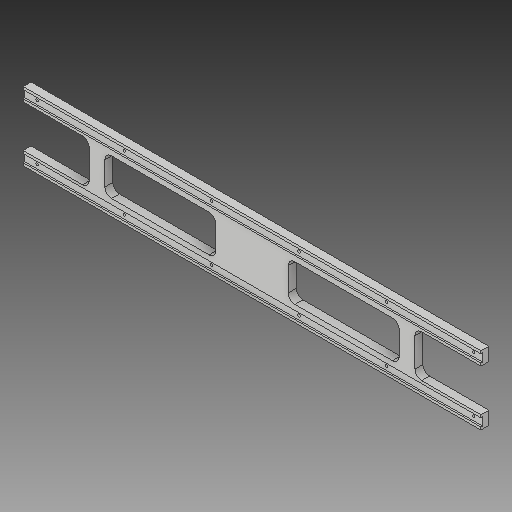
# Autodesk Inventor part: DriveTrainTop
Saved by Autodesk Inventor 2017 (Build 210142000, 142)
## iProperties
Created: 2016-10-18
Part Number: DriveTrainTop
Material: Generic
Document SubType Name: Sheet Metal
Designer: aesen
Density: 1 g/cm^3
Sheet Metal Rule: Default_mm
Appearance: Default
Author: aesen
Autodesk Inventor part; units mm, degrees
ref_plane "YZ Plane" through (0, 0, 0) normal (1, 0, 0) x (0, 1, 0)
ref_plane "XZ Plane" through (0, 0, 0) normal (0, 1, 0) x (-1, 0, 0)
ref_plane "XY Plane" through (0, 0, 0) normal (0, 0, 1) x (1, 0, 0)
sketch "Sketch1" plane through (0, 0, 0) normal (0, 0, 1) x (1, 0, 0)
  line L0 (-115.57, 41.275) -> (435.2925, 41.275)
  line L1 (435.2925, -41.275) -> (-115.57, -41.275)
  line L2 (422, 41.275) -> (422, 25.4)
  line L3 (424, -41.275) -> (424, -25.4)
  line L4 (355.9175, 17.4) -> (355.9175, -17.4)
  line L5 (355.9175, 6) -> (336.8675, 6)
  line L6 (321, 41.275) -> (321, 22.225)
  line L7 (322, -41.275) -> (322, -22.225)
  line L8 (336.8675, 14.225) -> (336.8675, -14.225)
  line L9 (-36.195, -17.4) -> (-36.195, 17.4)
  line L10 (-36.195, 0) -> (-17.145, 0)
  line L11 (-17.145, 14.225) -> (-17.145, -14.225)
  line L12 (-9.145, -22.225) -> (108.205, -22.225)
  line L13 (116.205, -14.225) -> (116.205, 14.225)
  line L14 (108.205, 22.225) -> (-9.145, 22.225)
  line L15 (116.205, 12) -> (203.518, 12)
  line L16 (211.518, 22.225) -> (328.8675, 22.225)
  line L17 (203.518, 14.225) -> (203.518, -14.225)
  line L18 (211.518, -22.225) -> (328.8675, -22.225)
  arc A0 (-9.145, 22.225) -> (-17.145, 14.225) centre (-9.145, 14.225) ccw
  arc A1 (116.205, 14.225) -> (108.205, 22.225) centre (108.205, 14.225) ccw
  arc A2 (-17.145, -14.225) -> (-9.145, -22.225) centre (-9.145, -14.225) ccw
  arc A3 (108.205, -22.225) -> (116.205, -14.225) centre (108.205, -14.225) ccw
  arc A4 (211.518, 22.225) -> (203.518, 14.225) centre (211.518, 14.225) ccw
  arc A5 (336.8675, 14.225) -> (328.8675, 22.225) centre (328.8675, 14.225) ccw
  arc A6 (328.8675, -22.225) -> (336.8675, -14.225) centre (328.8675, -14.225) ccw
  arc A7 (203.518, -14.225) -> (211.518, -22.225) centre (211.518, -14.225) ccw
  arc A8 (363.9175, 25.4) -> (355.9175, 17.4) centre (363.9175, 17.4) ccw
  arc A9 (355.9175, -17.4) -> (363.9175, -25.4) centre (363.9175, -17.4) ccw
  arc A10 (-36.195, 17.4) -> (-44.195, 25.4) centre (-44.195, 17.4) ccw
  arc A11 (-44.195, -25.4) -> (-36.195, -17.4) centre (-44.195, -17.4) ccw
  line L19 (435.2925, -41.275) -> (435.2925, 38.1)
  line L20 (-115.57, 41.275) -> (-115.57, -38.1)
  line L21 (-44.195, 25.4) -> (-115.57, 25.4)
  line L22 (-44.195, -25.4) -> (-115.57, -25.4)
  line L23 (363.9175, 25.4) -> (435.2925, 25.4)
  line L24 (363.9175, -25.4) -> (435.2925, -25.4)
  line L25 (-115.57, -38.1) -> (-115.57, -41.275)
  line L26 (435.2925, 41.275) -> (435.2925, 38.1)
  point P0 (0, 0)
  point P1 (0, 0)
  point P2 (-36.195, 25.4)
  point P3 (154, 41.275)
  point P4 (157.175, 41.275)
  point P5 (154, -41.275)
  point P6 (157.175, -41.275)
  dimension "d0" = 15.875
  dimension "d1" = 15.875
  dimension "d2" = 19.05
  dimension "d3" = 19.05
  dimension "d4" = 19.05
  dimension "d5" = 19.05
  dimension "d6" = 44.45
  dimension "d7" = 133.35
  dimension "d8" = 87.313
  dimension "d9" = 133.3495
  dimension "d10" = 8
  dimension "d11" = 79.375
  dimension "d12" = 79.375
  dimension "d13" = 550.8625
  constraints: 54 end point, 24 point on circle, 20 tangent, 15 point on line, 12 centre point, 11 equal radius, 9 perpendicular, 8 vertical, 5 horizontal, 2 parallel, 1 midpoint
  measures "d0" distance of L2.start L2.end
  measures "d1" distance of L3.end L3.start
  measures "d2" distance of L5.start L5.end
  measures "d3" distance of L6.start L6.end
  measures "d4" distance of L7.end L7.start
  measures "d5" distance of L10.start L10.end
  measures "d6" distance between parallel lines of L12 L14
  measures "d7" distance between parallel lines of L13 L11
  measures "d8" distance of L15.end L15.start
  measures "d9" distance between parallel lines of L8 L17
  measures "d10" radius of A0
  measures "d11" distance between parallel lines of L19 L4
  measures "d12" distance between parallel lines of L20 L9
  measures "d13" distance between parallel lines of L19 L20
extrude "Extrusion1" add sketch "Sketch1" along normal mid plane 9.525 contours L0 L6 L16 A4 L17 L15 L13 A1 L14 A0 L11 L10 L9 A10 L21 L20 | L0 L2 L23 A8 L4 L5 L8 A5 L16 L6 | L0 L26 L19 L23 L2 | L22 A11 L9 L10 L11 A2 L12 A3 L13 L15 L17 A7 L18 L7 L1 L25 L20 | L19 L1 L3 L24 | L5 L4 A9 L24 L3 L1 L7 L18 A6 L8
sketch "Sketch2" plane through (0, 0, 4.7625) normal (0, 0, 1) x (1, 0, 0)
  line L0 (-115.57, 41.275) -> (154, 41.275)
  line L1 (-71.7405, 41.275) -> (-71.7405, 38.1)
  line L2 (-44.195, 25.4) -> (-115.57, 25.4)
  line L3 (-83, 25.4) -> (-83, 28.575)
  line L4 (154, -41.275) -> (-130.57, -41.275)
  line L5 (-85, -41.275) -> (-85, -38.1)
  line L6 (-115.57, -25.4) -> (-44.195, -25.4)
  line L7 (-76, -25.4) -> (-76, -28.575)
  line L8 (-115.57, 25.4) -> (-115.57, 41.275)
  line L9 (435.2925, 25.4) -> (435.2925, 38.1)
  line L10 (-115.57, 38.1) -> (435.2925, 38.1)
  line L11 (435.2925, 38.1) -> (435.2925, 28.575)
  line L12 (435.2925, 28.575) -> (-115.57, 28.575)
  line L13 (-115.57, 28.575) -> (-115.57, 38.1)
  line L14 (-115.57, -38.1) -> (-115.57, -25.4)
  line L15 (435.2925, -25.4) -> (435.2925, -41.275)
  line L16 (-115.57, -28.575) -> (435.2925, -28.575)
  line L17 (435.2925, -28.575) -> (435.2925, -38.1)
  line L18 (435.2925, -38.1) -> (-115.57, -38.1)
  line L19 (-115.57, -38.1) -> (-115.57, -28.575)
  point P0 (0, 0)
  point P1 (0, 0)
  dimension "d16" = 3.175
  dimension "d17" = 3.175
  dimension "d18" = 3.175
  dimension "d19" = 3.175
  constraints: 40 end point, 8 point on line, 4 parallel, 3 perpendicular, 3 vertical, 2 horizontal
  measures "d16" distance of L1.start L1.end
  measures "d17" distance of L3.end L3.start
  measures "d18" distance of L5.end L5.start
  measures "d19" distance of L7.start L7.end
emboss "Emboss1" sketch "Sketch2" operation cut depth 2 direction (0, 0, -1) contours L10 L9 L12 L8 | L16 L15 L18 L14
sketch "Sketch3" plane through (0, 0, 4.7625) normal (0, 0, 1) x (1, 0, 0)
  circle A0 centre (4.2538, 33.3375) radius 3.175
  circle A1 centre (4.2538, -33.3375) radius 3.175
  circle A2 centre (-100.8387, 33.3375) radius 3.175
  circle A3 centre (-100.8387, -33.3375) radius 3.175
  circle A4 centre (109.3463, 33.3375) radius 3.175
  circle A5 centre (214.4388, 33.3375) radius 3.175
  circle A6 centre (319.5313, 33.3375) radius 3.175
  circle A7 centre (424.6238, 33.3375) radius 3.175
  circle A8 centre (109.3463, -33.3375) radius 3.175
  circle A9 centre (214.4388, -33.3375) radius 3.175
  circle A10 centre (319.5313, -33.3375) radius 3.175
  circle A11 centre (424.6238, -33.3375) radius 3.175
  point P0 (0, 0)
  point P1 (321.7538, 0)
  dimension "d22" = 6.35
  dimension "d23" = 6.35
  dimension "d24" = 6.35
  dimension "d25" = 6.35
  dimension "d26" = 6.35
  dimension "d27" = 6.35
  dimension "d28" = 6.35
  dimension "d29" = 6.35
  dimension "d30" = 6.35
  dimension "d31" = 6.35
  dimension "d32" = 6.35
  dimension "d33" = 6.35
  constraints: 12 centre point
  measures "d22" diameter of A0
  measures "d23" diameter of A2
  measures "d24" diameter of A3
  measures "d25" diameter of A4
  measures "d26" diameter of A1
  measures "d27" diameter of A8
  measures "d28" diameter of A5
  measures "d29" diameter of A9
  measures "d30" diameter of A6
  measures "d31" diameter of A10
  measures "d32" diameter of A7
  measures "d33" diameter of A11
hole "Hole2" at (-100.8387, -33.3375, 4.7625) at (109.3463, -33.3375, 4.7625) at (4.2538, -33.3375, 4.7625) at (214.4388, -33.3375, 4.7625) at (424.6238, -33.3375, 4.7625) at (424.6238, 33.3375, 4.7625) at (319.5313, 33.3375, 4.7625) at (319.5313, -33.3375, 4.7625) at (214.4388, 33.3375, 4.7625) at (109.3463, 33.3375, 4.7625) at (4.2538, 33.3375, 4.7625) at (-100.8387, 33.3375, 4.7625) direction (0, 0, -1) diameter 3 end through all countersink diameter 4 countersink angle 90
equation "\"d46\" = Thickness"
equation "\"BendRadius\" = Thickness"
equation "\"BendReliefWidth\" = Thickness"
equation "\"BendReliefDepth\" = 0.5 * Thickness"
equation "\"CornerReliefSize\" = 4 * Thickness"
equation "\"MinimumRemnant\" = 2 * Thickness"
equation "\"TransitionRadius\" = BendRadius"
equation "\"JacobiRadiusSize\" = BendRadius"
equation "\"GapSize\" = Thickness"
equation "\"Thickness\" = 0.5"
body "Solid1"
